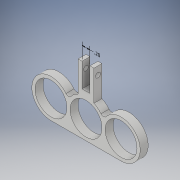
# Autodesk Inventor part: beta_dummy
Saved by Autodesk Inventor 2018 (Build 220112000, 112)
## iProperties
Created: 2017-10-07
Part Number: beta_dummy
Material: Generic
Document SubType Name: Modeling
Designer: rheal
Density: 1 g/cm^3
Appearance: Default
Author: rheal
Autodesk Inventor part; units mm, degrees
ref_plane "YZ Plane" through (0, 0, 0) normal (1, 0, 0) x (0, 1, 0)
ref_plane "XZ Plane" through (0, 0, 0) normal (0, 1, 0) x (-1, 0, 0)
ref_plane "XY Plane" through (0, 0, 0) normal (0, 0, 1) x (1, 0, 0)
sketch "Sketch1" plane through (0, 0, 0) normal (0, 0, 1) x (1, 0, 0)
  line L0 (-2.5, 10) -> (-2.5, 20)
  line L1 (2.5, 10) -> (2.5, 25)
  line L2 (2.5, 25) -> (5, 25)
  arc A0 (6.0006, 0.0769) -> (6, -0.0245) centre (14, -0.0245) ccw
  line L3 (-2.5, 10) -> (2.5, 10)
  line L4 (-5, 20) -> (-5, 5.9087)
  line L5 (0, 10) -> (0, 17.0552) construction
  line L6 (5, 25) -> (5, 5.9087)
  circle A1 centre (0, -5) radius 10
  line L7 (0, -5) -> (-38, -5) construction
  arc A2 (-5, 5.9087) -> (-9.4286, 2.4231) centre (0, -5) ccw
  arc A3 (12, -5) -> (22, -15) centre (22, -5) ccw
  arc A4 (9.4286, 2.4231) -> (5, 5.9087) centre (0, -5) ccw
  line L8 (0, -17) -> (22, -17)
  circle A5 centre (-22, -5) radius 10
  arc A6 (-12.5714, 2.4231) -> (-22, -17) centre (-22, -5) ccw
  arc A7 (-12.5714, 2.4231) -> (-9.4286, 2.4231) centre (-11, 3.6603) ccw
  line L9 (-22, -17) -> (0, -17)
  circle A8 centre (22, -5) radius 10
  arc A9 (22, -17) -> (12.5714, 2.4231) centre (22, -5) ccw
  arc A10 (9.4286, 2.4231) -> (12.5714, 2.4231) centre (11, 3.6603) ccw
  line L10 (-2.5, 20) -> (-2.5, 25)
  line L11 (-2.5, 25) -> (-5, 25)
  line L12 (-5, 25) -> (-5, 20)
  point P0 (0, 0)
  point P1 (8, 0)
  point P2 (-32, -5)
  point P3 (-12, -5)
  point P4 (-34, -5)
  point P5 (32, -5)
  point P6 (11, -9.7958)
  point P7 (-5, -15.9087)
  point P8 (38, -5)
  point P9 (32, -5)
  point P10 (34, -5)
  dimension "d12" = 2.5
  dimension "d13" = 10
  dimension "d14" = 2.5
  dimension "d15" = 15
  dimension "d24" = 20
  dimension "d36" = 2
  dimension "d44" = 5
  constraints: 26 end point, 16 point on circle, 11 centre point, 11 symmetric about line, 4 point on line, 3 coincident, 3 horizontal, 3 vertical, 2 perpendicular, 2 tangent, 1 midpoint, 3 other
  measures "d12" distance of L4.start L0.end
  measures "d13" distance of L0.end L0.start
  measures "d14" distance of L1.end L2.end
  measures "d15" distance of L1.start L1.end
  measures "d24" diameter of A1
  measures "d36" radius of A7
  measures "d44" distance of L0.start L1.start
extrude "Extrusion1" add sketch "Sketch1" along normal blind 5
sketch "Sketch3" plane through (0, 0, 5) normal (0, 0, 1) x (1, 0, 0)
  circle A0 centre (0, -5) radius 10
  point P0 (0, 0)
  dimension "d26" = 20
  constraints: 1 centre point
  measures "d26" diameter of A0
extrude "Extrusion3" cut sketch "Sketch3" against normal blind 5
fillet "Fillet2" [suppressed]
sketch "Sketch4" plane through (5, 5.9087, 0) normal (1, 0, 0) x (0, 0, -1)
  line L0 (0, 19.0913) -> (-5, 19.0913) construction
  line L1 (-2.5, 19.0913) -> (-2.5, 14.0913) construction
  circle A0 centre (-2.5, 14.0913) radius 1.5
  point P0 (0, -5.9087)
  dimension "d30" = 5
  dimension "d31" = 3
  constraints: 2 end point, 1 centre point, 1 coincident, 1 midpoint, 1 vertical
  measures "d30" distance of L1.start L1.end
  measures "d31" diameter of A0
extrude "Extrusion4" cut sketch "Sketch4" against normal blind 10
body "Solid1"
